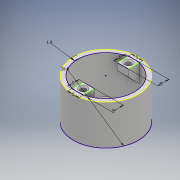
# Autodesk Inventor part: Clock Dot
Saved by Autodesk Inventor 2018 (Build 220112000, 112)
## iProperties
Created: 2021-04-21
Part Number: Clock Dot
Material: Generic
Document SubType Name: Modeling
Designer: Kevin
Density: 1 g/cm^3
Appearance: Default
Author: Kevin
Autodesk Inventor part; units mm, degrees
ref_plane "YZ Plane" through (0, 0, 0) normal (1, 0, 0) x (0, 1, 0)
ref_plane "XZ Plane" through (0, 0, 0) normal (0, 1, 0) x (-1, 0, 0)
ref_plane "XY Plane" through (0, 0, 0) normal (0, 0, 1) x (1, 0, 0)
sketch "Sketch10" plane through (0, 0, 0) normal (0, 0, 1) x (1, 0, 0)
  circle A0 centre (0, 0) radius 14.3
  dimension "d33" = 28.6
  constraints: 1 centre point, 1 coincident
  measures "d33" diameter of A0
extrude "Extrusion6" add sketch "Sketch10" along normal blind 17.6
sketch "Sketch11" plane through (0, 0, 17.6) normal (0, 0, 1) x (1, 0, 0)
  circle A0 centre (0, 0) radius 12.5
  circle A1 centre (0, 0) radius 14.3 projected
  dimension "d36" = 1.8
  constraints: 1 centre point, 1 coincident
  measures "d36" radial gap between concentric circles of A0 A1
extrude "Extrusion7" cut sketch "Sketch11" against normal blind 17 contours A0
sketch "Sketch12" plane through (0, 0, 17.6) normal (0, 0, 1) x (1, 0, 0)
  circle A0 centre (0, 0) radius 12.5 projected
  line L0 (2.5, 7.5) -> (-2.5, 7.5)
  line L1 (-2.5, 7.5) -> (-2.5, 12.5)
  line L2 (-2.5, 12.5) -> (2.5, 12.5)
  line L3 (2.5, 12.5) -> (2.5, 7.5)
  line L4 (2.5, -7.5) -> (-2.5, -7.5)
  line L5 (-2.5, -7.5) -> (-2.5, -12.5)
  line L6 (-2.5, -12.5) -> (2.5, -12.5)
  line L7 (2.5, -12.5) -> (2.5, -7.5)
  dimension "d41" = 5
  dimension "d42" = 5
  dimension "d43" = 5
  dimension "d46" = 5
  dimension "d47" = 5
  dimension "d48" = 5
  constraints: 16 end point, 4 parallel, 2 horizontal, 2 perpendicular
  measures "d41" distance of L1.end L2.end
  measures "d42" distance of L0.end L1.end
  measures "d43" distance edge to line of A0 L0
  measures "d46" distance of L6.end L5.end
  measures "d47" distance of L5.end L4.end
  measures "d48" distance edge to line of A0 L4
extrude "Extrusion8" add sketch "Sketch12" against normal blind 8 contours L3 L0 L1 A0 | A0 L2 L3 | L7 L6 A0 | A0 L5 L4 L7 | A0 L1 L2 | L6 L5 A0
sketch "Sketch18" plane through (2.5, 7.5, 17.6) normal (1, 0, 0) x (0, 0, -1)
  line L0 (0, 4.7474) -> (0, 0) projected
  line L1 (0, 0) -> (3, 0)
  line L2 (0, 0) -> (8, 0) projected
  line L3 (8, 5) -> (8, 4.7474) projected
  line L4 (3, 0) -> (8, 4.7474)
  line L5 (8, 4.7474) -> (8, 0)
  line L6 (8, 0) -> (3, 0)
  line L7 (0, -15) -> (8, -15) projected
  line L8 (0, -15) -> (3, -15)
  line L9 (0, -19.7474) -> (8, -19.7474) projected
  line L10 (3, -15) -> (8, -19.7474)
  line L11 (8, -19.7474) -> (8, -15)
  line L12 (8, -15) -> (3, -15)
  point P0 (17.6, -7.5)
  dimension "d56" = 3
  dimension "d57" = 3
  constraints: 16 end point, 4 perpendicular, 2 point on line
  measures "d56" distance of L0.end L1.end
  measures "d57" distance of L7.start L8.end
extrude "Extrusion9" cut sketch "Sketch18" against normal blind 5
sketch "Sketch19" plane through (0, 0, 17.6) normal (0, 0, 1) x (1, 0, 0)
  line L0 (2.5, 7.5) -> (-2.5, 7.5) projected
  arc A0 (2.5, 12.2474) -> (-2.5, 12.2474) centre (0, 0) ccw projected
  line L1 (-2.5, 7.5) -> (-2.5, 12.2474) projected
  line L2 (2.5, -7.5) -> (-2.5, -7.5) projected
  line L3 (-2.5, -7.5) -> (-2.5, -12.2474) projected
  point P0 (0, 10)
  point P1 (0, -10)
  dimension "d60" = 2.5
  dimension "d61" = 2.5
  dimension "d63" = 2.5
  dimension "d64" = 2.5
  measures "d60" distance from line of L1 point (0, 10)
  measures "d61" distance from line of L0 point (0, 10)
  measures "d63" distance from line of L2 point (0, -10)
  measures "d64" distance from line of L3 point (0, -10)
hole "Hole2" at (0, 10, 17.6) at (0, -10, 17.6) direction (0, 0, -1) diameter 2.4 depth 10 tip angle 118
chamfer "Chamfer2" distance 0.6 angle 45 2 edges at (0, -8.8, 17.6) (0, 11.2, 17.6)
body "Solid2"
